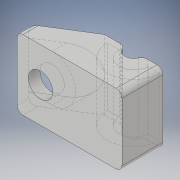
# Autodesk Inventor part: passe cable
Saved by Autodesk Inventor 2019 (Build 230136000, 136)
## iProperties
Created: 2019-02-11
Part Number: passe cable
Material: Générique
Document SubType Name: Modeling
Designer: xavier
Density: 1 g/cm^3
Appearance: Par défaut
Author: xavier
Autodesk Inventor part; units mm, degrees
ref_plane "YZ Plane" through (0, 0, 0) normal (1, 0, 0) x (0, 1, 0)
ref_plane "XZ Plane" through (0, 0, 0) normal (0, 1, 0) x (-1, 0, 0)
sketch "Esquisse1" plane through (0, 0, 0) normal (0, 0, 1) x (1, 0, 0)
  line L0 (0, 0) -> (8, 0)
  line L1 (8, 0) -> (8, 12)
  line L2 (8, 12) -> (0, 12)
  line L3 (0, 12) -> (0, 0)
  dimension "d0" = 8
  dimension "d1" = 12
  constraints: 8 end point, 2 parallel, 1 horizontal, 1 perpendicular
  measures "d0" distance of L2.end L1.end
  measures "d1" distance of L1.end L0.end
extrude "Extrusion1" add sketch "Esquisse1" along normal blind 2
sketch "Esquisse2" plane through (0, 0, 2) normal (0, 0, 1) x (1, 0, 0)
  line L0 (8, 0) -> (8, 12) projected
  line L1 (8, 12) -> (18, 12)
  line L2 (18, 12) -> (18, 0)
  line L3 (18, 0) -> (8, 0)
  line L4 (8, 0) -> (8, 12)
  point P0 (0, 0)
  dimension "d7" = 10
  constraints: 8 end point, 2 parallel, 1 horizontal, 1 perpendicular
  measures "d7" distance of L2.end L3.end
extrude "Extrusion2" add sketch "Esquisse2" against normal blind 7
chamfer "Chanfrein1" distance 5 distance2 8 1 edges at (8, 6, 0) measured on face at (8, 4, -1.6667)
sketch "Esquisse3" plane through (0, 0, -5) normal (0, 0, -1) x (-1, 0, 0)
  arc A0 (-4, 10) -> (-4, 2) centre (-4, 6) ccw
  line L0 (-8, 0) -> (-8, 12) projected
  line L1 (-4, 2) -> (4, 2)
  line L2 (4, 2) -> (4, 10)
  line L3 (4, 10) -> (-4, 10)
  point P0 (0, 0)
  dimension "d13" = 8
  constraints: 6 end point, 2 point on circle, 1 centre point, 1 horizontal, 1 parallel, 1 perpendicular, 1 tangent
  measures "d13" diameter of A0
extrude "Extrusion3" cut sketch "Esquisse3" against normal blind 5
sketch "Esquisse4" plane through (0, 0, 0) normal (0, 0, -1) x (-1, 0, 0)
  arc A0 (-4, 10) -> (-8, 6) centre (-4, 6) ccw projected
  circle A1 centre (-4, 6) radius 2.1
  point P0 (0, 0)
  dimension "d16" = 4.2
  constraints: 1 centre point, 1 coincident
  measures "d16" diameter of A1
extrude "Extrusion4" cut sketch "Esquisse4" against normal through all
ref_plane "Plan de construction2" through (0, 6, 2) normal (0, 1, 0) x (1, 0, 0)
sketch "Esquisse10" plane through (0, 6, 2) normal (0, 1, 0) x (1, 0, 0)
  line L0 (18, 7) -> (8, 7) projected
  circle A0 centre (13, 7) radius 3.5
  point P0 (0, 2)
  dimension "d29" = 7
  constraints: 1 centre point, 1 midpoint
  measures "d29" diameter of A0
sketch "Esquisse12" plane through (0, 0, -5) normal (0, 0, -1) x (-1, 0, 0)
  line L0 (-9.5, 6) -> (-16.5, 6) projected
  line L1 (-8.5, 11) -> (-10.5, 11)
  line L2 (-10.5, 11) -> (-10.5, 1)
  line L3 (-10.5, 1) -> (-8.5, 1)
  line L4 (-8.5, 1) -> (-8.5, 11)
  line L5 (-8.5, 11) -> (-10.5, 1) construction
  line L6 (-10.5, 11) -> (-8.5, 1) construction
  point P0 (0, 0)
  dimension "d30" = 2
  constraints: 12 end point, 2 midpoint, 2 parallel, 1 horizontal, 1 perpendicular
  measures "d30" distance of L3.end L2.end
sweep "Balayage2" cut profiles "Esquisse12" path "Esquisse10" path curves A0
sketch "Esquisse13" plane through (0, 6, 2) normal (0, 1, 0) x (1, 0, 0)
  line L0 (8, 7) -> (18, 7) projected
  circle A0 centre (13, 7) radius 1.5
  point P0 (0, 2)
  dimension "d33" = 3
  constraints: 1 centre point, 1 midpoint
  measures "d33" diameter of A0
extrude "Extrusion6" cut sketch "Esquisse13" along normal through all both and the other way through all
fillet "Congé3" radius 1 4 edges at (14.5, 3, -5) (14.5, 9, -5) (11.5, 9, -5) (11.5, 3, -5)
fillet "Congé4" radius 1 4 edges at (18, 12, -1.5) (18, 0, -1.5) (0, 0, 1) (0, 12, 1)
